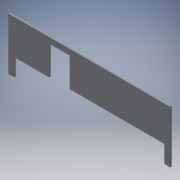
# Autodesk Inventor part: SmallWall
Saved by Autodesk Inventor 2017 (Build 210142000, 142)
## iProperties
Created: 2017-03-24
Part Number: SmallWall
Material: Generic
Document SubType Name: Modeling
Designer: hoeflinc
Density: 1 g/cm^3
Appearance: Default
Quantity: 1
Author: hoeflinc
Autodesk Inventor part; units mm, degrees
ref_plane "YZ Plane" through (0, 0, 0) normal (1, 0, 0) x (0, 1, 0)
ref_plane "XZ Plane" through (0, 0, 0) normal (0, 1, 0) x (-1, 0, 0)
ref_plane "XY Plane" through (0, 0, 0) normal (0, 0, 1) x (1, 0, 0)
sketch "Sketch1" plane through (0, 0, 0) normal (0, 0, 1) x (1, 0, 0)
  line L0 (0, 0) -> (352.425, 0)
  line L1 (352.425, 0) -> (352.425, 114.3)
  line L2 (352.425, 114.3) -> (0, 114.3)
  line L3 (0, 114.3) -> (0, 0)
  dimension "d0" = 352.425
  dimension "d1" = 114.3
  constraints: 8 end point, 2 parallel, 1 horizontal, 1 perpendicular
  measures "d0" distance of L0.start L0.end
  measures "d1" distance of L2.end L0.start
extrude "Extrusion1" add sketch "Sketch1" along normal blind 3.175
sketch "Sketch2" plane through (0, 0, 3.175) normal (0, 0, 1) x (1, 0, 0)
  line L0 (12.7, 0) -> (339.725, 0)
  line L1 (339.725, 0) -> (339.725, 38.1)
  line L2 (339.725, 38.1) -> (12.7, 38.1)
  line L3 (12.7, 38.1) -> (12.7, 0)
  line L4 (0, 114.3) -> (0, 0) projected
  line L5 (352.425, 0) -> (352.425, 114.3) projected
  dimension "d4" = 12.7
  dimension "d5" = 12.7
  dimension "d6" = 38.1
  constraints: 8 end point, 2 parallel, 1 horizontal, 1 perpendicular
  measures "d4" distance between parallel lines of L4 L3
  measures "d5" distance between parallel lines of L1 L5
  measures "d6" distance of L2.end L0.start
extrude "Extrusion2" cut sketch "Sketch2" against normal blind 25.4
sketch "Sketch3" plane through (0, 0, 3.175) normal (0, 0, 1) x (1, 0, 0)
  line L0 (339.725, 38.1) -> (12.7, 38.1) projected
  line L1 (88.9, 38.1) -> (133.35, 38.1)
  line L2 (133.35, 38.1) -> (133.35, 101.6)
  line L3 (133.35, 101.6) -> (88.9, 101.6)
  line L4 (88.9, 101.6) -> (88.9, 38.1)
  point P0 (0, 0)
  dimension "d9" = 63.5
  dimension "d10" = 76.2
  dimension "d11" = 44.45
  constraints: 8 end point, 2 parallel, 1 horizontal, 1 perpendicular, 1 point on line
  measures "d9" distance of L3.end L1.start
  measures "d10" distance from line of L0.end L4
  measures "d11" distance of L2.end L3.end
extrude "Extrusion3" cut sketch "Sketch3" against normal blind 25.4
body "Solid1"
